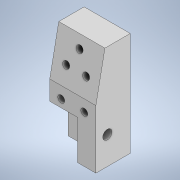
# Autodesk Inventor part: connector
Saved by Autodesk Inventor 2020 (Build 240168000, 168)
## iProperties
Created: 2019-06-19
Part Number: connector
Material: Generic
Document SubType Name: Modeling
Designer: Vivek Muskan
Density: 1 g/cm^3
Appearance: Default
Author: Vivek Muskan
Autodesk Inventor part; units mm, degrees
ref_plane "YZ Plane" through (0, 0, 0) normal (1, 0, 0) x (0, 1, 0)
ref_plane "XZ Plane" through (0, 0, 0) normal (0, 1, 0) x (-1, 0, 0)
ref_plane "XY Plane" through (0, 0, 0) normal (0, 0, 1) x (1, 0, 0)
sketch "Sketch1" plane through (0, 0, 0) normal (1, 0, 0) x (0, 1, 0)
  line L0 (0, 0) -> (19.6116, -3.9223)
  line L1 (0, 0) -> (20, 0) construction
  line L2 (19.6116, -3.9223) -> (19.6116, -14.9223)
  line L3 (19.6116, -14.9223) -> (-10.3884, -14.9223)
  line L4 (-10.3884, -14.9223) -> (-10.3884, 0)
  line L5 (-10.3884, 0) -> (0, 0)
  dimension "d0" = 20
  dimension "d1" = 11.31
  dimension "d2" = 11
  dimension "d3" = 30
  constraints: 12 end point, 3 perpendicular, 1 equal length, 1 horizontal, 1 vertical
  measures "d0" distance of L0.start L0.end
  measures "d1" angle of L0 L1
  measures "d2" distance of L0.end L2.end
  measures "d3" distance of L2.end L3.end
extrude "Extrusion1" add sketch "Sketch1" along normal blind 20
sketch "Sketch2" plane through (0, 0, 0) normal (0, 0.1961, 0.9806) x (1, 0, 0)
  line L0 (0, 0) -> (10, 0)
  line L1 (0, 0) -> (20, 0) projected
  line L2 (10, 0) -> (10, 15)
  circle A0 centre (10, 15) radius 1.5
  line L3 (10, 15) -> (10, 10)
  circle A1 centre (5.6699, 7.5) radius 1.5
  circle A2 centre (14.3301, 7.5) radius 1.5
  dimension "d6" = 15
  dimension "d7" = 3
  dimension "d8" = 5
  dimension "d11" = 360
  constraints: 6 end point, 3 centre point, 1 coincident, 1 midpoint, 1 perpendicular, 1 point on line, 7 other
  measures "d6" distance of L0.end L2.end
  measures "d7" diameter of A0
  measures "d8" distance of L3.start L3.end
extrude "Extrusion2" cut sketch "Sketch2" against normal blind 20
sketch "Sketch3" plane through (0, -10.3884, 0) normal (0, 0, 1) x (1, 0, 0)
  line L0 (0, 10.3884) -> (0, 0) projected
  line L1 (0, 10.3884) -> (0, 5.3884)
  line L2 (0, 5.3884) -> (5, 5.3884)
  line L3 (5, 5.3884) -> (15, 5.3884)
  circle A0 centre (5, 5.3884) radius 1.5
  circle A1 centre (15, 5.3884) radius 1.5
  dimension "d15" = 5
  dimension "d16" = 5
  dimension "d17" = 10
  dimension "d18" = 3
  dimension "d19" = 3
  constraints: 6 end point, 2 centre point, 2 coincident, 1 horizontal, 1 perpendicular, 1 point on line
  measures "d15" distance of L0.start L1.end
  measures "d16" distance of L1.end L2.end
  measures "d17" distance of L2.end L3.end
  measures "d18" diameter of A0
  measures "d19" diameter of A1
extrude "Extrusion3" cut sketch "Sketch3" against normal blind 20
sketch "Sketch4" plane through (20, 0, 0) normal (1, 0, 0) x (0, 0, -1)
  line L0 (14.9223, -10.3884) -> (14.9223, 19.6116) projected
  line L1 (0, -10.3884) -> (14.9223, -10.3884) projected
  line L2 (14.9223, -10.3884) -> (0, -10.3884)
  point P0 (0, 0)
  constraints: 2 end point, 1 horizontal
sketch "Sketch5" plane through (20, 0, 0) normal (1, 0, 0) x (0, 0, -1)
  line L0 (0, 0) -> (0, -10.3884) projected
  line L1 (0, -10.3884) -> (14.9223, -10.3884)
  line L2 (14.9223, -10.3884) -> (14.9223, -25.3884)
  line L3 (14.9223, -25.3884) -> (0, -25.3884)
  line L4 (0, -25.3884) -> (0, -10.3884)
  dimension "d22" = 15
  dimension "d25" = 14.9223
  constraints: 8 end point, 2 parallel, 1 horizontal, 1 perpendicular
  measures "d22" distance of L1.end L2.end
  measures "d25" distance of L2.end L3.end
extrude "Extrusion4" add sketch "Sketch5" against normal blind 20
sketch "Sketch10" plane through (0, 0, 0) normal (0, 0, 1) x (1, 0, 0)
  line L0 (0, -25.3884) -> (0, 19.6116) projected
  line L1 (0, -25.3884) -> (12, -25.3884)
  line L2 (12, -25.3884) -> (12, -8.3884)
  line L3 (12, -8.3884) -> (0, -8.3884)
  line L4 (0, -8.3884) -> (0, -25.3884)
  point P0 (0, 0)
  point P1 (0, -8.3884)
  dimension "d39" = 12
  dimension "d40" = 17
  constraints: 8 end point, 2 parallel, 1 horizontal, 1 perpendicular
  measures "d39" distance of L3.end L2.end
  measures "d40" distance of L2.end L1.end
extrude "Extrusion8" cut sketch "Sketch10" against normal blind 8
sketch "Sketch11" plane through (20, 0, 0) normal (1, 0, 0) x (0, 0, -1)
  line L0 (0, -25.3884) -> (8, -25.3884) projected
  line L1 (0, -25.3884) -> (5, -25.3884)
  line L2 (5, -25.3884) -> (5, -13.3884)
  circle A0 centre (5, -13.3884) radius 2
  point P0 (0, 0)
  dimension "d43" = 5
  dimension "d44" = 12
  dimension "d45" = 4
  constraints: 4 end point, 1 centre point, 1 coincident, 1 point on line, 1 vertical
  measures "d43" distance of L0.start L1.end
  measures "d44" distance of L1.end L2.end
  measures "d45" diameter of A0
extrude "Extrusion9" cut sketch "Sketch11" against normal blind 8
sketch "Sketch12" plane through (20, 19.6116, -14.9223) normal (0, 0, -1) x (-1, 0, 0)
  line L0 (20, -45) -> (20, 0) projected
  line L1 (20, -45) -> (13.5, -45)
  line L2 (8, -45) -> (20, -45) projected
  line L3 (13.5, -45) -> (13.5, -33)
  circle A0 centre (13.5, -33) radius 2
  point P0 (20, -19.6116)
  dimension "d48" = 6.5
  dimension "d49" = 12
  dimension "d50" = 4
  constraints: 4 end point, 1 centre point, 1 coincident, 1 perpendicular, 1 point on line
  measures "d48" distance of L0.start L1.end
  measures "d49" distance of L1.end L3.end
  measures "d50" diameter of A0
extrude "Extrusion10" cut sketch "Sketch12" against normal blind 8
body "Solid1"
